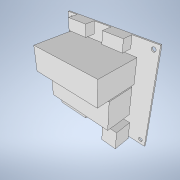
# Autodesk Inventor part: Плата
Saved by Autodesk Inventor 2021.1 (Build 251245010, 245A)
## iProperties
Created: 2026-06-28
Part Number: Плата
Material: Типовые
Document SubType Name: Modeling
Designer: Андрей Тарасов
Density: 1 g/cm^3
Appearance: По умолчанию
Author: Андрей Тарасов
Autodesk Inventor part; units mm, degrees
ref_plane "YZ Plane" through (0, 0, 0) normal (1, 0, 0) x (0, 1, 0)
ref_plane "XZ Plane" through (0, 0, 0) normal (0, 1, 0) x (-1, 0, 0)
ref_plane "XY Plane" through (0, 0, 0) normal (0, 0, 1) x (1, 0, 0)
sketch "Эскиз1" plane through (0, 0, 0) normal (0, 0, 1) x (1, 0, 0)
  line L0 (0, 0) -> (58, 0)
  line L1 (58, 0) -> (58, 60)
  line L2 (58, 60) -> (0, 60)
  line L3 (0, 60) -> (0, 0)
  line L4 (0, 57) -> (58, 57) construction
  line L5 (0, 3) -> (58, 3) construction
  line L6 (3, 0) -> (3, 60) construction
  line L7 (55, 60) -> (55, 0) construction
  circle A0 centre (3, 57) radius 1.25
  circle A1 centre (55, 57) radius 1.25
  circle A2 centre (55, 3) radius 1.25
  circle A3 centre (3, 3) radius 1.25
  dimension "d0" = 58
  dimension "d1" = 60
  dimension "d2" = 52
  dimension "d3" = 54
  dimension "d4" = 3
  dimension "d5" = 3
  dimension "d6" = 2.5
  constraints: 16 end point, 16 point on line, 4 centre point, 4 perpendicular, 3 equal radius, 3 parallel, 1 horizontal
  measures "d0" distance of L0.start L0.end
  measures "d1" distance of L2.end L0.start
  measures "d2" distance between parallel lines of L7 L6
  measures "d3" distance between parallel lines of L5 L4
  measures "d4" distance between parallel lines of L0 L5
  measures "d5" distance between parallel lines of L3 L6
  measures "d6" diameter of A0
extrude "Выдавливание1" add sketch "Эскиз1" along normal blind 1
sketch "Эскиз2" plane through (0, 0, 1) normal (0, 0, 1) x (1, 0, 0)
  line L0 (37, -2) -> (47, -2)
  line L1 (47, -2) -> (47, 10)
  line L2 (47, 10) -> (37, 10)
  line L3 (37, 10) -> (37, -2)
  line L4 (0, 60) -> (0, 0) projected
  line L5 (58, 0) -> (58, 60) projected
  line L6 (0, 0) -> (58, 0) projected
  dimension "d9" = 37
  dimension "d10" = 11
  dimension "d14" = 2
  dimension "d15" = 12
  constraints: 8 end point, 2 parallel, 1 horizontal, 1 perpendicular
  measures "d9" distance between parallel lines of L3 L4
  measures "d10" distance between parallel lines of L5 L1
  measures "d14" distance between parallel lines of L6 L0
  measures "d15" distance between parallel lines of L2 L0
extrude "Выдавливание2" add sketch "Эскиз2" along normal blind 11
sketch "Эскиз3" plane through (0, 0, 1) normal (0, 0, 1) x (1, 0, 0)
  line L0 (7, 60) -> (19.5, 60)
  line L1 (19.5, 60) -> (19.5, 53)
  line L2 (19.5, 53) -> (7, 53)
  line L3 (7, 53) -> (7, 60)
  line L4 (58, 60) -> (0, 60) projected
  line L5 (0, 60) -> (0, 0) projected
  line L6 (58, 0) -> (58, 60) projected
  line L7 (30.5, 60) -> (43, 60)
  line L8 (43, 60) -> (43, 53)
  line L9 (43, 53) -> (30.5, 53)
  line L10 (30.5, 53) -> (30.5, 60)
  dimension "d16" = 7
  dimension "d18" = 15
  dimension "d19" = 12.5
  dimension "d20" = 7
  constraints: 16 end point, 4 collinear, 4 parallel, 2 horizontal, 2 perpendicular
  measures "d16" distance between parallel lines of L3 L5
  measures "d18" distance between parallel lines of L6 L8
  measures "d19" distance of L8.end L9.end
  measures "d20" distance of L7.end L8.end
extrude "Выдавливание3" add sketch "Эскиз3" along normal blind 6
sketch "Эскиз4" plane through (0, 0, 1) normal (0, 0, 1) x (1, 0, 0)
  line L0 (3, 50) -> (47, 50)
  line L1 (47, 50) -> (47, 35)
  line L2 (47, 35) -> (3, 35)
  line L3 (3, 35) -> (3, 50)
  line L4 (0, 60) -> (0, 0) projected
  line L5 (30.5, 60) -> (19.5, 60) projected
  dimension "d23" = 15
  dimension "d24" = 44
  dimension "d25" = 3
  dimension "d26" = 10
  constraints: 8 end point, 2 parallel, 1 horizontal, 1 perpendicular
  measures "d23" distance of L2.end L0.start
  measures "d24" distance of L0.start L0.end
  measures "d25" distance between parallel lines of L3 L4
  measures "d26" distance between parallel lines of L0 L5
extrude "Выдавливание4" add sketch "Эскиз4" along normal blind 26
sketch "Эскиз5" plane through (0, 0, 1) normal (0, 0, 1) x (1, 0, 0)
  line L0 (3, 33) -> (46, 33)
  line L1 (46, 33) -> (46, 15)
  line L2 (46, 15) -> (3, 15)
  line L3 (3, 15) -> (3, 33)
  line L4 (0, 0) -> (37, 0) projected
  line L5 (0, 60) -> (0, 0) projected
  line L6 (58, 0) -> (58, 60) projected
  dimension "d29" = 15
  dimension "d30" = 3
  dimension "d31" = 18
  dimension "d32" = 12
  constraints: 8 end point, 2 parallel, 1 horizontal, 1 perpendicular
  measures "d29" distance between parallel lines of L4 L2
  measures "d30" distance between parallel lines of L3 L5
  measures "d31" distance of L2.end L0.start
  measures "d32" distance between parallel lines of L6 L1
extrude "Выдавливание5" add sketch "Эскиз5" along normal blind 17
sketch "Эскиз6" plane through (0, 0, 1) normal (0, 0, 1) x (1, 0, 0)
  line L0 (24, 12) -> (3, 12)
  line L1 (3, 12) -> (3, 6)
  line L2 (3, 6) -> (24, 6)
  line L3 (24, 6) -> (24, 12)
  line L4 (0, 0) -> (37, 0) projected
  line L5 (0, 60) -> (0, 0) projected
  dimension "d35" = 6
  dimension "d36" = 3
  dimension "d37" = 6
  dimension "d38" = 21
  constraints: 8 end point, 2 parallel, 1 horizontal, 1 perpendicular
  measures "d35" distance between parallel lines of L4 L2
  measures "d36" distance between parallel lines of L5 L1
  measures "d37" distance of L0.end L1.end
  measures "d38" distance of L0.start L0.end
extrude "Выдавливание6" add sketch "Эскиз6" along normal blind 11
